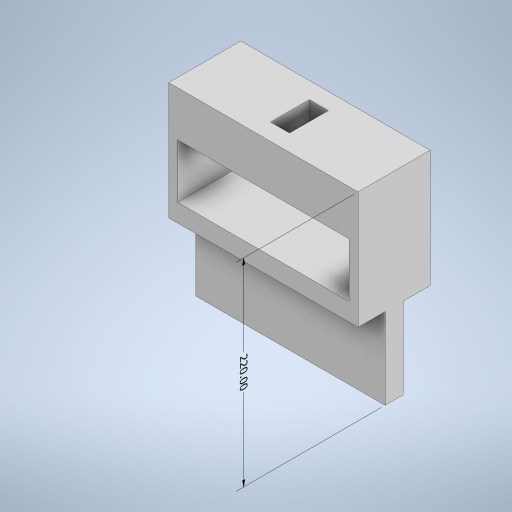
# Autodesk Inventor part: front_support
Saved by Autodesk Inventor 2023 (Build 270158000, 158)
## iProperties
Created: 2022-10-31
Part Number: front_support
Material: Genérico
Document SubType Name: Modeling
Designer: papel
Density: 1 g/cm^3
Appearance: Valor por defecto
Author: papel
Autodesk Inventor part; units mm, degrees
ref_plane "YZ Plane" through (0, 0, 0) normal (1, 0, 0) x (0, 1, 0)
ref_plane "XY Plane" through (0, 0, 0) normal (0, 0, 1) x (1, 0, 0)
sketch "Boceto1" plane through (0, 0, 0) normal (0, 1, 0) x (-1, 0, 0)
  line L0 (105, 40) -> (-105, 40)
  line L1 (-105, 40) -> (-105, -40)
  line L2 (-105, -40) -> (105, -40)
  line L3 (105, -40) -> (105, 40)
  line L4 (105, 40) -> (-105, -40) construction
  line L5 (-105, 40) -> (105, -40) construction
  point P0 (0, 0)
  dimension "d0" = 210
  dimension "d1" = 80
  constraints: 12 end point, 2 midpoint, 2 parallel, 1 horizontal, 1 perpendicular
  measures "d0" distance of L2.end L1.end
  measures "d1" distance of L1.end L0.end
extrude "Extrusión1" add sketch "Boceto1" along normal blind 130
sketch "Boceto2" plane through (-105, 0, 40) normal (0, 0, 1) x (1, 0, 0)
  line L0 (10, 80) -> (200, 80)
  line L1 (200, 80) -> (200, 20)
  line L2 (200, 20) -> (10, 20)
  line L3 (10, 20) -> (10, 80)
  line L4 (10, 80) -> (200, 20) construction
  line L5 (200, 80) -> (10, 20) construction
  line L6 (0, 0) -> (210, 0) projected
  point P0 (105, 0)
  point P1 (105, 50)
  dimension "d4" = 190
  dimension "d5" = 60
  dimension "d6" = 20
  constraints: 12 end point, 2 midpoint, 2 parallel, 1 horizontal, 1 perpendicular
  measures "d4" distance of L1.end L2.end
  measures "d5" distance of L0.end L1.end
  measures "d6" distance between parallel lines of L6 L2
extrude "Extrusión2" cut sketch "Boceto2" against normal blind 60
sketch "Boceto3" plane through (0, 130, 0) normal (0, 1, 0) x (1, 0, 0)
  line L0 (-10.5, -21.5) -> (10.5, -21.5)
  line L1 (10.5, -21.5) -> (10.5, 21.5)
  line L2 (10.5, 21.5) -> (-10.5, 21.5)
  line L3 (-10.5, 21.5) -> (-10.5, -21.5)
  line L4 (-10.5, -21.5) -> (10.5, 21.5) construction
  line L5 (10.5, -21.5) -> (-10.5, 21.5) construction
  point P0 (0, 0)
  point P1 (0, 0)
  dimension "d9" = 21
  dimension "d10" = 43
  constraints: 12 end point, 2 midpoint, 2 parallel, 1 horizontal, 1 perpendicular
  measures "d9" distance of L2.end L1.end
  measures "d10" distance of L1.end L0.end
extrude "Extrusión3" cut sketch "Boceto3" against normal blind 43
sketch "Boceto4" plane through (0, 0, 0) normal (0, -1, 0) x (1, 0, 0)
  line L0 (105, 40) -> (105, -40) projected
  line L1 (-105, 10) -> (105, 10)
  line L2 (105, 10) -> (105, -10)
  line L3 (105, -10) -> (-105, -10)
  line L4 (-105, -10) -> (-105, 10)
  line L5 (-105, 10) -> (105, -10) construction
  line L6 (105, 10) -> (-105, -10) construction
  point P0 (0, 0)
  dimension "d13" = 20
  constraints: 12 end point, 2 midpoint, 2 parallel, 1 horizontal, 1 perpendicular, 1 point on line
  measures "d13" distance of L1.end L2.end
extrude "Extrusión4" add sketch "Boceto4" along normal blind 90
ref_plane "Plano de trabajo1" through (0, -90, 0) normal (0, 1, 0) x (-1, 0, 0)
sketch "Boceto7" plane through (0, -90, 0) normal (0, 1, 0) x (-1, 0, 0)
  circle A0 centre (11.5239, -60) radius 3
  circle A1 centre (-11.4761, -60) radius 3
  line L0 (105, 10) -> (-105, 10)
  line L1 (105.0239, -10) -> (-104.9761, -10)
  line L2 (105.0239, -10) -> (-104.9761, -10)
  circle A2 centre (11.5239, -30) radius 3
  circle A3 centre (-11.4761, -30) radius 3
  line L3 (11.5239, -60) -> (-11.4761, -30)
  line L4 (11.5239, -30) -> (-11.4761, -60)
  line L5 (105, 10) -> (-105, 10)
  line L6 (-105, 10) -> (-95.8154, 10)
  line L7 (0.0239, -45) -> (-34.9761, -45)
  line L8 (0.0239, -45) -> (35.0239, -45)
  line L9 (35.0239, -45) -> (35.0239, -10)
  line L10 (-105, -10) -> (105, -10)
  line L11 (35.0239, -10) -> (-34.9761, -10)
  line L12 (-34.9761, -10) -> (-34.9761, -79)
  line L13 (-34.9761, -79) -> (35.0239, -79)
  line L14 (35.0239, -79) -> (35.0239, -10)
  line L15 (-105, -10) -> (105, -10) projected
  line L16 (-40.6213, -10) -> (-84.6707, -10)
  point P0 (0, 0)
  point P1 (0, 0)
  point P2 (0.0478, -10)
  dimension "d28" = 20
  dimension "d29" = 20
  dimension "d30" = 30
  dimension "d31" = 30
  dimension "d32" = 20
  dimension "d33" = 35
  dimension "d34" = 35
  dimension "d35" = 69
  constraints: 32 end point, 4 centre point, 4 point on line, 3 equal length, 3 horizontal, 2 perpendicular, 1 midpoint
  measures "d28" distance from line of L1 A2.centre
  measures "d29" distance from line of A3.centre L1
  measures "d30" distance between centres of A1 A3
  measures "d31" distance of A0.centre A2.centre
  measures "d32" distance between parallel lines of L0 L1
  measures "d33" distance of L8.start L7.end
  measures "d34" distance of L8.start L8.end
  measures "d35" distance of L13.start L12.start
extrude "Extrusión6" add sketch "Boceto7" along normal blind 10 separate body
ref_plane "Plano de trabajo3" through (-0.0239, -90, -79) normal (-1, 0, 0) x (0, 0, 1)
sketch "Boceto10" plane through (-0.0239, -90, -79) normal (-1, 0, 0) x (0, 0, 1)
  line L0 (57.1622, 10) -> (81.4718, 10) construction
  line L1 (69, 33.1018) -> (55.6622, 10)
  line L2 (69, 33.1018) -> (69, 10)
  line L3 (69, 90) -> (69, 0) projected
  line L4 (0, 10) -> (69, 10) projected
  line L5 (69, 10) -> (55.6622, 10)
  point P0 (79, 90)
  dimension "d45" = 1.5
  constraints: 8 end point, 2 point on line, 1 collinear, 1 horizontal
  measures "d45" distance of L0.start L1.end
extrude "Extrusión7" add sketch "Boceto10" along normal mid plane 10 bodies 2
